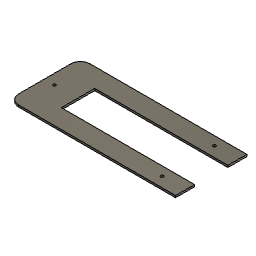
base v2 (Autodesk Fusion 360 design; units mm, degrees)
Autodesk Fusion 360 part; units mm, degrees
sketch "Sketch1" plane through (0, 0, 0) normal (0, 1, 0) x (1, 0, 0)
  line L0 (140, -17.5) -> (-140, -17.5)
  line L1 (-140, -17.5) -> (-140, 17.5)
  line L2 (-140, 17.5) -> (140, 17.5)
  line L3 (140, 17.5) -> (140, -17.5)
  line L4 (140, -17.5) -> (-140, 17.5) construction
  line L5 (-140, -17.5) -> (140, 17.5) construction
  line L6 (150, -27.5) -> (-150, -27.5)
  line L7 (-150, -27.5) -> (-150, 27.5)
  line L8 (-150, 27.5) -> (150, 27.5)
  line L9 (150, 27.5) -> (150, -27.5)
  line L10 (150, -27.5) -> (-150, 27.5) construction
  line L11 (-150, -27.5) -> (150, 27.5) construction
  dimension "d1" = 280
  dimension "d2" = 35
  dimension "d3" = 300
  dimension "d4" = 55
  constraint horizontal L0
  constraint perpendicular L0 L1
  constraint parallel L0 L2
  constraint parallel L1 L3
  constraint coincident L4 origin
  constraint coincident L5 origin
  constraint horizontal L6
  constraint perpendicular L6 L7
  constraint parallel L6 L8
  constraint parallel L7 L9
  constraint coincident L10 origin
  constraint coincident L11 origin
  measures "d1" distance of L1.end L2.end
  measures "d2" distance of L0.end L1.end
  measures "d3" distance of L7.end L8.end
  measures "d4" distance of L6.end L7.end
extrude "Extrude1" add sketch "Sketch1" along normal blind 2
sketch "Sketch2" plane through (0, 0, 27.5) normal (0, 0, 1) x (1, 0, 0)
  line L0 (-150, 0) -> (150, 0)
  line L1 (150, 0) -> (150, 2)
  line L2 (150, 2) -> (-150, 2)
  line L3 (-150, 2) -> (-150, 0)
extrude "Extrude2" add sketch "Sketch2" along normal blind 20
move_face "OffsetFaces1" offset 25 1 faces at (-150, 0.6667, 22.5)
sketch "Sketch3" plane through (0, 0, 0) normal (0, 1, 0) x (1, 0, 0)
  line L0 (155, -50) -> (0, -50)
  line L1 (0, -50) -> (0, 50)
  line L2 (0, 50) -> (155, 50)
  line L3 (155, 50) -> (155, -50)
  constraint horizontal L0
  constraint vertical L1
  constraint horizontal L2
  constraint vertical L3
extrude "Extrude3" cut sketch "Sketch3" along normal blind 60
fillet "Fillet1" radius 10 1 edges at (-175, 1, 47.5)
fillet "Fillet2" radius 10 1 edges at (-175, 1, -27.5)
move_face "OffsetFaces2" offset -10 1 faces at (-46.6667, 0.6667, 17.5)
move_face "OffsetFaces3" offset 10 1 faces at (-93.3333, 0.6667, -17.5)
hole "Hole1" at (-164.3594, 2, 10.5834) direction (0, -1, 0) diameter 3 depth 5 tip angle 118
hole "Hole2" at (-24.6611, 2, 36.9776) direction (0, -1, 0) diameter 3 depth 5 tip angle 118
hole "Hole3" at (-24.9224, 2, -18.284) direction (0, -1, 0) diameter 3 depth 5 tip angle 118
